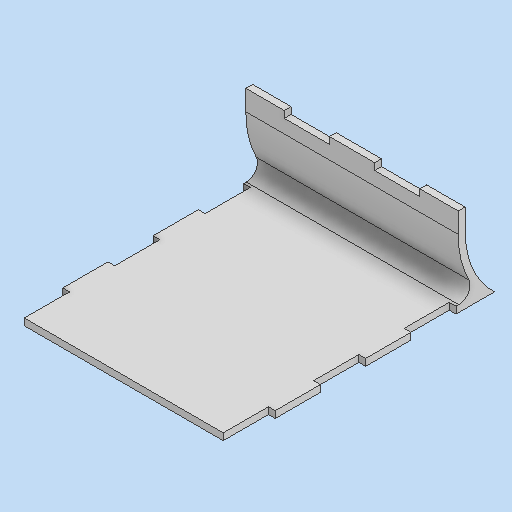
# Autodesk Inventor part: bridge plate
Saved by Autodesk Inventor 2026 (Build 300175000, 175)
## iProperties
Created: 2026-02-15
Part Number: bridge plate
Material: Generic
Document SubType Name: Modeling
Designer: mones
Density: 1 g/cm^3
Appearance: Default
Author: mones
Autodesk Inventor part; units mm, degrees
ref_plane "YZ Plane" through (0, 0, 0) normal (1, 0, 0) x (0, 1, 0)
ref_plane "XZ Plane" through (0, 0, 0) normal (0, 1, 0) x (-1, 0, 0)
ref_plane "XY Plane" through (0, 0, 0) normal (0, 0, 1) x (1, 0, 0)
sketch "Sketch1" plane through (0, 0, 0) normal (1, 0, 0) x (0, 1, 0)
  arc A0 (16.4511, -26.4081) -> (-13.5489, -39.4081) centre (16.4011, -67.4081) ccw
  line L0 (22.4511, -26.4081) -> (16.4511, -26.4081)
  line L1 (-13.5489, 77.5919) -> (-13.5489, -39.4081)
  line L2 (-10.5489, 77.5919) -> (-10.5489, -32.6274)
  arc A1 (16.4529, -23.4081) -> (-10.5489, -32.6274) centre (16.4011, -67.4081) ccw
  line L3 (16.4529, -23.4081) -> (22.4511, -23.4081)
  line L4 (-10.5489, 77.5919) -> (-13.5489, 77.5919)
  line L5 (22.4511, -23.4081) -> (22.4511, -26.4081)
  dimension "d0" = 3
  constraints: 12 end point, 4 point on circle, 2 centre point, 2 perpendicular, 2 other
  measures "d0" radial gap between concentric circles of A0 A1
extrude "Extrusion1" add sketch "Sketch1" along normal blind 94
sketch "Sketch2" plane through (0, 0, 0) normal (-1, 0, 0) x (0, 0, 1)
  line L0 (-32.6274, -10.5489) -> (77.5919, -10.5489) projected
  arc A0 (-32.6274, -10.5489) -> (-23.4081, 16.4529) centre (-67.4081, 16.4011) ccw projected
  line L1 (-23.4081, 22.4511) -> (-23.4081, 16.4529) projected
  line L2 (-26.4081, 22.4511) -> (-23.4081, 22.4511) projected
  line L3 (-26.4081, 16.4511) -> (-26.4081, 22.4511) projected
  arc A1 (-39.4081, -13.5489) -> (-26.4081, 16.4511) centre (-67.4081, 16.4011) ccw projected
  line L4 (77.5919, -13.5489) -> (-39.4081, -13.5489) projected
  line L5 (77.5919, -10.5489) -> (77.5919, -13.5489) projected
  line L6 (77.5919, -10.5489) -> (57.5919, -10.5489)
  line L7 (57.5919, -10.5489) -> (37.5919, -10.5489)
  line L8 (37.5919, -10.5489) -> (17.5919, -10.5489)
  line L9 (17.5919, -10.5489) -> (-2.4081, -10.5489)
  line L10 (-2.4081, -10.5489) -> (-22.4081, -10.5489)
  line L11 (-22.4081, -10.5489) -> (-22.4081, -13.5489)
  line L12 (-2.4081, -10.5489) -> (-2.4081, -13.5489)
  line L13 (17.5919, -10.5489) -> (17.5919, -13.5489)
  line L14 (37.5919, -10.5489) -> (37.5919, -13.5489)
  line L15 (57.5919, -10.5489) -> (57.5919, -13.5489)
  line L16 (77.5919, -13.5489) -> (-22.4081, -13.5489)
  line L17 (77.5919, -10.5489) -> (-22.4081, -10.5489)
  dimension "d3" = 20
  dimension "d4" = 20
  dimension "d5" = 20
  dimension "d6" = 20
  dimension "d7" = 20
  constraints: 24 end point, 10 point on line, 2 collinear, 2 parallel, 2 perpendicular, 1 vertical
  measures "d3" distance of L0.end L6.end
  measures "d4" distance of L6.end L7.end
  measures "d5" distance of L7.end L8.end
  measures "d6" distance of L8.end L9.end
  measures "d7" distance of L9.end L10.end
extrude "Extrusion2" cut sketch "Sketch2" against normal blind 3 contours L0 L12 L4 L11 | L0 L14 L4 L13 | L0 L5 L4 L15
sketch "Sketch3" plane through (94, 0, 0) normal (1, 0, 0) x (0, 0, -1)
  line L0 (32.6274, -10.5489) -> (-77.5919, -10.5489) projected
  line L1 (-77.5919, -10.5489) -> (-77.5919, -13.5489) projected
  line L2 (-77.5919, -13.5489) -> (39.4081, -13.5489) projected
  arc A0 (26.4081, 16.4511) -> (39.4081, -13.5489) centre (67.4081, 16.4011) ccw projected
  line L3 (26.4081, 16.4511) -> (26.4081, 22.4511) projected
  line L4 (26.4081, 22.4511) -> (23.4081, 22.4511) projected
  line L5 (23.4081, 22.4511) -> (23.4081, 16.4529) projected
  arc A1 (23.4081, 16.4529) -> (32.6274, -10.5489) centre (67.4081, 16.4011) ccw projected
  line L6 (-77.5919, -13.5489) -> (-57.5919, -13.5489)
  line L7 (-57.5919, -13.5489) -> (-37.5919, -13.5489)
  line L8 (-37.5919, -13.5489) -> (-17.5919, -13.5489)
  line L9 (-17.5919, -13.5489) -> (2.4081, -13.5489)
  line L10 (2.4081, -13.5489) -> (22.4081, -13.5489)
  line L11 (22.4081, -13.5489) -> (22.4081, -10.5489)
  line L12 (2.4081, -13.5489) -> (2.4081, -10.5489)
  line L13 (-17.5919, -13.5489) -> (-17.5919, -10.5489)
  line L14 (-37.5919, -13.5489) -> (-37.5919, -10.5489)
  line L15 (-57.5919, -10.5489) -> (-57.5919, -13.5489)
  line L16 (-77.5919, -10.5489) -> (22.4081, -10.5489)
  line L17 (-77.5919, -13.5489) -> (22.4081, -13.5489)
  dimension "d10" = 20
  dimension "d11" = 20
  dimension "d12" = 20
  dimension "d13" = 20
  dimension "d14" = 20
  constraints: 24 end point, 10 point on line, 3 perpendicular, 2 collinear, 1 parallel, 1 vertical
  measures "d10" distance of L1.end L6.end
  measures "d11" distance of L6.end L7.end
  measures "d12" distance of L7.end L8.end
  measures "d13" distance of L8.end L9.end
  measures "d14" distance of L9.end L10.end
extrude "Extrusion3" cut sketch "Sketch3" against normal blind 3 contours L11 L2 L12 L0 | L13 L2 L14 L0 | L15 L2 L1 L0
sketch "Sketch4" plane through (0, 22.4511, -23.4081) normal (0, 1, 0) x (1, 0, 0)
  line L0 (0, 3) -> (0, 0) projected
  line L1 (0, 0) -> (94, 0) projected
  line L2 (94, 3) -> (94, 0) projected
  line L3 (0, 3) -> (94, 3) projected
  line L4 (94, 3) -> (0, 3)
  line L5 (94, 3) -> (67, 3)
  line L6 (67, 3) -> (55, 3)
  line L7 (55, 3) -> (43, 3)
  line L8 (43, 3) -> (31, 3)
  line L9 (31, 3) -> (19, 3)
  line L10 (19, 3) -> (0, 3)
  line L11 (67, 3) -> (47, 3)
  line L12 (47, 3) -> (67, 3)
  line L13 (47, 3) -> (27, 3)
  line L14 (94, 3) -> (77, 3)
  line L15 (77, 3) -> (57, 3)
  line L16 (57, 3) -> (37, 3)
  line L17 (37, 3) -> (17, 3)
  line L18 (17, 3) -> (17, 0)
  line L19 (37, 3) -> (37, 0)
  line L20 (57, 3) -> (57, 0)
  line L21 (77, 3) -> (77, 0)
  line L22 (0, 0) -> (0, 3)
  line L23 (94, 0) -> (94, 3)
  line L24 (94, 0) -> (0, 0)
  line L25 (94, 3) -> (0, 3)
  dimension "d26" = 17
  dimension "d27" = 20
  dimension "d28" = 20
  dimension "d29" = 20
  constraints: 44 end point, 14 point on line, 4 collinear, 3 parallel, 3 perpendicular, 2 midpoint
  measures "d26" distance of L2.start L14.end
  measures "d27" distance of L14.end L15.end
  measures "d28" distance of L15.end L16.end
  measures "d29" distance of L16.end L17.end
extrude "Extrusion4" add sketch "Sketch4" along normal blind 3 contours L3 L18 L1 L0 | L19 L3 L20 L1 | L21 L3 L2 L1
fillet "Fillet1" radius 5 1 edges at (47, -10.5489, -32.6274)
body "Solid1"
